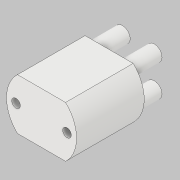
# Autodesk Inventor part: Caster_wheel_inner_plug_2_02
Saved by Autodesk Inventor 2019.3 (Build 233278000, 278)
## iProperties
Created: 2019-03-27
Part Number: Caster_wheel_inner_plug_2_02
Material: Generic
Document SubType Name: Modeling
Designer: Varga Daniel
Density: 1 g/cm^3
Appearance: White - P 1-1 C
Author: Varga Daniel
Autodesk Inventor part; units mm, degrees
ref_plane "YZ Plane" through (0, 0, 0) normal (1, 0, 0) x (0, 1, 0)
ref_plane "XZ Plane" through (0, 0, 0) normal (0, 1, 0) x (-1, 0, 0)
ref_plane "XY Plane" through (0, 0, 0) normal (0, 0, 1) x (1, 0, 0)
sketch "Sketch1" plane through (0, 0, 0) normal (0, 0, 1) x (1, 0, 0)
  arc A0 (0.6966, -35.7262) -> (5.6966, -30.7262) centre (0.6966, -30.7262) ccw
  line L0 (5.6966, -30.7262) -> (5.6966, -0.7262)
  arc A1 (5.6966, -0.7262) -> (0.6966, 4.2738) centre (0.6966, -0.7262) ccw
  line L1 (0.6966, 4.2738) -> (-29.3034, 4.2738)
  arc A2 (-29.3034, 4.2738) -> (-34.3034, -0.7262) centre (-29.3034, -0.7262) ccw
  line L2 (-34.3034, -0.7262) -> (-34.3034, -30.7262)
  arc A3 (-34.3034, -30.7262) -> (-29.3034, -35.7262) centre (-29.3034, -30.7262) ccw
  line L3 (-29.3034, -35.7262) -> (0.6966, -35.7262)
  line L4 (4.6966, -0.7262) -> (4.6966, -30.7262)
  arc A4 (0.6966, -34.7262) -> (4.6966, -30.7262) centre (0.6966, -30.7262) ccw
  line L5 (0.6966, -34.7262) -> (-3.8034, -34.7262)
  line L6 (-3.8034, 3.2738) -> (0.6966, 3.2738)
  arc A5 (4.6966, -0.7262) -> (0.6966, 3.2738) centre (0.6966, -0.7262) ccw
  line L7 (-4.8034, -34.7262) -> (-13.8034, -34.7262)
  line L8 (-13.8034, 3.2738) -> (-4.8034, 3.2738)
  line L9 (-14.8034, -34.7262) -> (-23.8034, -34.7262)
  line L10 (-23.8034, 3.2738) -> (-14.8034, 3.2738)
  line L11 (-33.3034, -30.7262) -> (-33.3034, -0.7262)
  arc A6 (-29.3034, 3.2738) -> (-33.3034, -0.7262) centre (-29.3034, -0.7262) ccw
  line L12 (-29.3034, 3.2738) -> (-24.8034, 3.2738)
  line L13 (-24.8034, -34.7262) -> (-29.3034, -34.7262)
  arc A7 (-33.3034, -30.7262) -> (-29.3034, -34.7262) centre (-29.3034, -30.7262) ccw
  circle A8 centre (-19.3034, -20.7262) radius 2.5
  circle A9 centre (-19.3034, -10.7262) radius 2.5
  circle A10 centre (-9.3034, -20.7262) radius 2.5
  circle A11 centre (-9.3034, -10.7262) radius 2.5
  circle A12 centre (-22.3034, -15.7262) radius 1.35
  circle A13 centre (-6.3034, -15.7262) radius 1.35
  line L14 (-21.8532, -23.7262) -> (-6.7536, -23.7262)
  circle A14 centre (-19.3034, -20.7262) radius 2.4
  circle A15 centre (-19.3034, -10.7262) radius 2.4
  circle A16 centre (-9.3034, -10.7262) radius 2.4
  circle A17 centre (-9.3034, -20.7262) radius 2.4
  arc A18 (-25.3034, -15.7262) -> (-21.8532, -23.7262) centre (-14.3034, -15.7262) ccw
  arc A19 (-6.7536, -23.7262) -> (-3.3034, -15.7262) centre (-14.3034, -15.7262) ccw
  line L15 (-25.3034, -15.7262) -> (-3.3034, -15.7262) construction
  line L16 (-6.7536, -7.7262) -> (-21.8532, -7.7262)
  arc A20 (-3.3034, -15.7262) -> (-6.7536, -7.7262) centre (-14.3034, -15.7262) ccw
  arc A21 (-21.8532, -7.7262) -> (-25.3034, -15.7262) centre (-14.3034, -15.7262) ccw
  line L17 (-23.8034, -34.7262) -> (-23.8034, -23.7262)
  line L18 (-24.8034, 3.2738) -> (-24.8034, -2.9057)
  line L19 (-24.8034, -23.7262) -> (-24.8034, -34.7262)
  line L20 (-4.8034, 3.2738) -> (-4.8034, -7.7262)
  line L21 (-4.8034, -23.7262) -> (-4.8034, -34.7262)
  line L22 (-3.8034, -34.7262) -> (-3.8034, -23.7262)
  line L23 (-3.8034, -7.7262) -> (-3.8034, 3.2738)
  circle A22 centre (-6.3034, -15.7262) radius 2
  circle A23 centre (-22.3034, -15.7262) radius 2
  point P0 (0, 0)
  dimension "d0" = 0.1
  dimension "d1" = 0.1
  dimension "d2" = 0.1
  dimension "d3" = 0.1
  dimension "d12" = 4
  dimension "d13" = 4
  dimension "d16" = 2.7
  constraints: 48 end point, 25 point on circle, 24 centre point, 6 point on line, 4 coincident, 2 parallel, 2 symmetric about line
  measures "d0" radial gap between concentric circles of A8 A14
  measures "d1" radial gap between concentric circles of A9 A15
  measures "d2" radial gap between concentric circles of A11 A16
  measures "d3" radial gap between concentric circles of A10 A17
  measures "d12" diameter of A23
  measures "d13" diameter of A22
  measures "d16" diameter of A13
extrude "Extrusion2" add sketch "Sketch1" along normal blind 21.23 contours A8 | A9 | A10 | A11 | A12 | A13 | A18 A21 L16 A20 A19 L14 | A14 | A15 | A16 | A17 | A22 | A23
extrude "Extrusion3" add sketch "Sketch1" against normal blind 9.2 contours A14 | A15 | A16 | A17
extrude "Extrusion4" cut sketch "Sketch1" along normal through all contours A12 | A13
extrude "Extrusion5" cut sketch "Sketch1" along normal blind 19.23 contours A22 | A23
equation "\"d13\" = d12"
equation "\"d6\" = inner_plug_height"
equation "\"inner_plug_height\" = 21.23"
body "Solid2"
